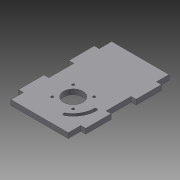
# Autodesk Inventor part: top
Saved by Autodesk Inventor 2015 (Build 190159000, 159)
## iProperties
Created: 2017-03-04
Part Number: top
Material: Generic
Document SubType Name: Modeling
Designer: Guy
Density: 1 g/cm^3
Appearance: Default
Author: Guy
Autodesk Inventor part; units mm, degrees
ref_plane "YZ Plane" through (0, 0, 0) normal (1, 0, 0) x (0, 1, 0)
ref_plane "XZ Plane" through (0, 0, 0) normal (0, 1, 0) x (-1, 0, 0)
ref_plane "XY Plane" through (0, 0, 0) normal (0, 0, 1) x (1, 0, 0)
sketch "Sketch1" plane through (0, 0, 0) normal (0, 0, 1) x (1, 0, 0)
  line L0 (0, 0) -> (120, 0)
  line L1 (120, 0) -> (120, 80)
  line L2 (120, 80) -> (0, 80)
  line L3 (0, 80) -> (0, 0)
  dimension "d0" = 120
  dimension "d1" = 80
  constraints: 8 end point, 2 parallel, 1 horizontal, 1 perpendicular
  measures "d0" distance of L2.end L1.end
  measures "d1" distance of L1.end L0.end
extrude "Extrusion1" add sketch "Sketch1" along normal blind 6
sketch "Sketch2" plane through (0, 0, 6) normal (0, 0, 1) x (1, 0, 0)
  line L0 (0, 0) -> (120, 0) projected
  line L1 (120, 0) -> (120, 80) projected
  line L2 (120, 80) -> (0, 80) projected
  line L3 (0, 80) -> (0, 0) projected
  line L4 (0, 80) -> (14.875, 80)
  line L5 (14.875, 80) -> (14.875, 74.125)
  line L6 (14.875, 74.125) -> (0, 74.125)
  line L7 (0, 74.125) -> (0, 80)
  line L8 (120, 80) -> (0, 80) projected
  line L9 (45.125, 80) -> (74.875, 80)
  line L10 (74.875, 80) -> (74.875, 74.125)
  line L11 (74.875, 74.125) -> (45.125, 74.125)
  line L12 (45.125, 74.125) -> (45.125, 80)
  line L13 (120, 80) -> (105.125, 80)
  line L14 (105.125, 80) -> (105.125, 74.125)
  line L15 (105.125, 74.125) -> (120, 74.125)
  line L16 (120, 74.125) -> (120, 80)
  line L17 (120, 0) -> (105.125, 0)
  line L18 (105.125, 0) -> (105.125, 5.875)
  line L19 (105.125, 5.875) -> (120, 5.875)
  line L20 (120, 5.875) -> (120, 0)
  line L21 (0, 0) -> (120, 0) projected
  line L22 (74.875, 0) -> (45.125, 0)
  line L23 (45.125, 0) -> (45.125, 5.875)
  line L24 (45.125, 5.875) -> (74.875, 5.875)
  line L25 (74.875, 5.875) -> (74.875, 0)
  line L26 (0, 0) -> (14.875, 0)
  line L27 (14.875, 0) -> (14.875, 5.875)
  line L28 (14.875, 5.875) -> (0, 5.875)
  line L29 (0, 5.875) -> (0, 0)
  line L30 (60, 104.1502) -> (60, -33.6862)
  line L31 (120, 0) -> (120, 80) projected
  dimension "d4" = 5.875
  dimension "d5" = 5.875
  dimension "d6" = 14.875
  dimension "d7" = 29.75
  dimension "d9" = 14.875
  dimension "d19" = 60
  dimension "d20" = 14.875
  constraints: 50 end point, 13 parallel, 7 point on line, 6 horizontal, 6 perpendicular, 3 collinear
  measures "d4" distance between parallel lines of L2 L6
  measures "d5" distance between parallel lines of L26 L28
  measures "d6" distance between parallel lines of L3 L5
  measures "d7" distance between parallel lines of L10 L12
  measures "d9" distance between parallel lines of L1 L14
  measures "d19" distance between parallel lines of L30 L1
  measures "d20" distance between parallel lines of L12 L30
extrude "Extrusion2" cut sketch "Sketch2" against normal up to next contours L3 L28 L27 L0 | L23 L24 L30 L0 | L3 L2 L5 L6 | L30 L24 L25 L0 | L18 L19 L1 L0 | L30 L2 L10 L11 | L11 L12 L2 L30 | L15 L14 L2 L1
sketch "Sketch4" plane through (0, 0, 6) normal (0, 0, 1) x (1, 0, 0)
  circle A0 centre (40, 40) radius 4.6
  line L0 (0, 74.125) -> (0, 5.875) projected
  line L1 (45.125, 80) -> (14.875, 80) projected
  point P0 (0, 0)
  dimension "d14" = 40
  dimension "d15" = 40
  dimension "d16" = 9.2
  constraints: 1 centre point
  measures "d14" distance from line of L0 A0.centre
  measures "d15" distance from line of A0.centre L1
  measures "d16" diameter of A0
extrude "Extrusion4" cut sketch "Sketch4" against normal up to next
sketch "Sketch5" plane through (0, 0, 6) normal (0, 0, 1) x (1, 0, 0)
  circle A0 centre (40, 40) radius 4.6 projected
  line L0 (74.875, 5.875) -> (74.875, 0) projected
  line L1 (74.875, 0) -> (105.125, 0) projected
  line L2 (105.125, 0) -> (105.125, 5.875) projected
  line L3 (105.125, 5.875) -> (120, 5.875) projected
  line L4 (120, 5.875) -> (120, 74.125) projected
  line L5 (120, 74.125) -> (105.125, 74.125) projected
  line L6 (105.125, 74.125) -> (105.125, 80) projected
  line L7 (105.125, 80) -> (74.875, 80) projected
  line L8 (74.875, 80) -> (74.875, 74.125) projected
  line L9 (74.875, 74.125) -> (45.125, 74.125) projected
  line L10 (45.125, 74.125) -> (45.125, 80) projected
  line L11 (45.125, 80) -> (14.875, 80) projected
  line L12 (14.875, 80) -> (14.875, 74.125) projected
  line L13 (14.875, 74.125) -> (0, 74.125) projected
  line L14 (0, 74.125) -> (0, 5.875) projected
  line L15 (0, 5.875) -> (14.875, 5.875) projected
  line L16 (14.875, 5.875) -> (14.875, 0) projected
  line L17 (14.875, 0) -> (45.125, 0) projected
  line L18 (45.125, 0) -> (45.125, 5.875) projected
  line L19 (45.125, 5.875) -> (74.875, 5.875) projected
  line L20 (52.5, 27.5) -> (27.5, 27.5)
  line L21 (27.5, 27.5) -> (27.5, 52.5)
  line L22 (27.5, 52.5) -> (52.5, 52.5)
  line L23 (52.5, 52.5) -> (52.5, 27.5)
  circle A1 centre (40, 40) radius 11.5
  circle A2 centre (52.5, 27.5) radius 1.5
  circle A3 centre (27.5, 27.5) radius 1.5
  circle A4 centre (27.5, 52.5) radius 1.5
  circle A5 centre (52.5, 52.5) radius 1.5
  circle A6 centre (40, 40) radius 26.387 construction
  line L24 (40, 40) -> (40, 13.613) construction
  line L25 (40, 40) -> (17.1482, 26.8065) construction
  arc A7 (40, 11.613) -> (40, 15.613) centre (40, 13.613) ccw
  arc A8 (18.8802, 27.8065) -> (15.4161, 25.8065) centre (17.1482, 26.8065) ccw
  arc A9 (18.8802, 27.8065) -> (40, 15.613) centre (40, 40) ccw
  arc A10 (15.4161, 25.8065) -> (40, 11.613) centre (40, 40) ccw
  point P0 (0, 0)
  dimension "d21" = 3
  dimension "d22" = 3
  dimension "d23" = 3
  dimension "d24" = 3
  dimension "d25" = 23
  dimension "d26" = 25
  dimension "d27" = 25
  dimension "d28" = 12.5
  dimension "d29" = 12.5
  dimension "d30" = 52.774
  dimension "d31" = 60
  dimension "d32" = 4
  dimension "d33" = 4
  constraints: 12 end point, 10 centre point, 10 coincident, 10 point on circle, 2 parallel, 2 tangent, 1 horizontal, 1 perpendicular, 1 vertical
  measures "d21" diameter of A2
  measures "d22" diameter of A3
  measures "d23" diameter of A4
  measures "d24" diameter of A5
  measures "d25" diameter of A1
  measures "d26" distance of L22.end L20.start
  measures "d27" distance of L20.start L20.end
  measures "d28" distance from line of A1.centre L20
  measures "d29" distance from line of A0.centre L23
  measures "d30" diameter of A6
  measures "d31" angle of L24 L25
  measures "d32" diameter of A7
  measures "d33" diameter of A8
extrude "Extrusion5" cut sketch "Sketch5" against normal blind 10 contours A3 L21 L20 | L20 L21 A3 | A2 L23 L20 | L20 L23 A2 | A4 L22 L21 | L21 L22 A4 | A5 L22 L23 | L23 L22 A5 | A1 | A10 A8 A9 A7
equation "\"d22\" = d21"
equation "\"d23\" = d21"
equation "\"d24\" = d21"
equation "\"d28\" = 0.5 * d26"
equation "\"d29\" = 0.5 * d27"
body "Solid1"
